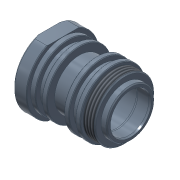
# Autodesk Inventor part: NA-45-h-Crown-307
Saved by Autodesk Inventor 2020.2 (Build 242310000, 310)
## iProperties
Created: 2020-04-21
Part Number: NA-45-h-Crown-307
Material: 14 100
Description: DRZAK CHYTAKU
Document SubType Name: Modeling
Designer: Jurek
Density: 7.85 g/cm^3
Mass: 123.312 g
Surface Area: 91.3308 cm^2
Volume: 15.7085 cm^3
Appearance: Ocelově modrá(1)
User Status: Rychlá změna
Checked By: Pippal
Category: B
Hmotnost (kg): 0,12
Rozmer_A: 36,7
Rozmer_B: 0
Rozmer_C: 0
Rozmer_D: 41
Rada vyrobku: 4100
Prumer nadobky: 45
Cislo artiklu: 4451101407
Jednotka: ks
Cisty rozmer: =Ø<Rozmer_A> - <Rozmer_D>
Predpona: Ø
Stroj na lince: Stahovací lis
RAZ Poznamka 1: ISO 2768-mH
RAZ Poznamka 2: NEOZNAČENÉ HRANY OJEHLIT
DXF: Ne
QAD_code: M
Rizeni davek: L
Author: Jurek
Revision Number: 00
Autodesk Inventor part; units mm, degrees
ref_plane "YZ Plane" through (0, 0, 0) normal (1, 0, 0) x (0, 1, 0)
ref_plane "XZ Plane" through (0, 0, 0) normal (0, 1, 0) x (-1, 0, 0)
ref_plane "XY Plane" through (0, 0, 0) normal (0, 0, 1) x (1, 0, 0)
sketch "Náčrt1" plane through (0, 0, 0) normal (0, 0, 1) x (1, 0, 0)
  line L0 (0, 0) -> (20.108, 0)
  line L1 (0, 12.5) -> (0, 18.35)
  line L2 (0, 18.35) -> (7, 18.35)
  line L3 (7, 18.35) -> (7, 16.35)
  line L4 (7, 16.35) -> (9.5, 16.35)
  line L5 (9.5, 16.35) -> (9.5, 14)
  line L6 (9.5, 14) -> (12.7, 14)
  line L7 (12.7, 14) -> (12.7, 16.35)
  line L8 (12.7, 16.35) -> (15.2, 16.35)
  line L9 (15.2, 16.35) -> (15.2, 12.5)
  line L10 (15.2, 12.5) -> (23.8, 12.5)
  line L11 (23.8, 12.5) -> (23.8, 16.35)
  line L12 (23.8, 16.35) -> (26.3, 16.35)
  line L13 (26.3, 16.35) -> (26.3, 14)
  line L14 (26.3, 14) -> (29.5, 14)
  line L15 (29.5, 14) -> (29.5, 16.35)
  line L16 (29.5, 16.35) -> (32, 16.35)
  line L17 (32, 16.35) -> (32, 15)
  line L18 (32, 15) -> (38, 15)
  line L19 (38, 15) -> (38, 12)
  line L20 (38, 12) -> (41, 12)
  line L21 (41, 12) -> (41, 10.2679)
  line L22 (40, 10) -> (34.5, 10)
  line L23 (33.567, 10.25) -> (10.933, 10.25)
  line L24 (10, 10) -> (2.5, 10)
  line L25 (34.5, 10) -> (33.567, 10.25)
  line L26 (10, 10) -> (10.933, 10.25)
  line L27 (0, 12.5) -> (2.5, 10)
  line L28 (40, 10) -> (41, 10.2679)
  dimension "d0" = 41
  dimension "d1" = 36.7
  dimension "d2" = 24
  dimension "d3" = 30
  dimension "d4" = 3
  dimension "d5" = 9
  dimension "d6" = 32.7
  dimension "d7" = 25
  dimension "d9" = 20
  dimension "d10" = 20
  dimension "d11" = 20.5
  dimension "d15" = 34
  dimension "d16" = 2.5
  dimension "d17" = 2.5
  dimension "d18" = 2.5
  dimension "d19" = 2.5
  dimension "d20" = 3.2
  dimension "d21" = 3.2
  dimension "d23" = 28
  dimension "d24" = 15
  dimension "d25" = 15
  dimension "d50" = 25
  dimension "d51" = 10
  dimension "d52" = 2.5
  dimension "d53" = 45
  dimension "d54" = 6.5
  dimension "d55" = 15
  dimension "d56" = 1
  constraints: 58 end point, 21 parallel, 5 point on line, 2 horizontal, 2 perpendicular
  measures "d0" distance between parallel lines of L21 L1
  measures "d1" diameter of L2 L0
  measures "d2" diameter of L20 L0
  measures "d3" diameter of L18 L0
  measures "d4" distance between parallel lines of L19 L21
  measures "d5" distance between parallel lines of L17 L21
  measures "d6" diameter of L16 L0
  measures "d7" diameter of L10 L0
  measures "d9" diameter of L24 L0
  measures "d10" diameter of L22 L0
  measures "d11" diameter of L23 L0
  measures "d15" distance between parallel lines of L3 L21
  measures "d16" distance between parallel lines of L15 L17
  measures "d17" distance between parallel lines of L11 L13
  measures "d18" distance between parallel lines of L7 L9
  measures "d19" distance between parallel lines of L5 L3
  measures "d20" distance between parallel lines of L15 L13
  measures "d21" distance between parallel lines of L7 L5
  measures "d23" diameter of L14 L0
  measures "d24" angle of L26 L24
  measures "d25" angle of L25 L22
  measures "d50" distance between parallel lines of L17 L3
  measures "d51" distance from line of L24.start L1
  measures "d52" distance from line of L24.end L1
  measures "d53" angle of L27 L24
  measures "d54" distance from line of L22.end L21
  measures "d55" angle of L28 L22
  measures "d56" distance from line of L22.start L21
revolve "Rotace1" add sketch "Náčrt1" angle 360 about axis through (0, 0, 0) along (1, 0, 0)
chamfer "Zkosení1" distance 1 angle 45 1 edges at (0, -18.35, 0)
chamfer "Zkosení2" distance 0.3 angle 45 1 edges at (7, -18.35, 0)
chamfer "Zkosení3" distance 0.5 angle 45 1 edges at (41, -12, 0)
chamfer "Zkosení4" distance 0.3 angle 45 7 edges at (32, -16.35, 0) (29.5, -16.35, 0) (26.3, -16.35, 0) (23.8, -16.35, 0) (15.2, -16.35, 0) (12.7, -16.35, 0) (9.5, -16.35, 0)
thread "Závit1" size "M30x1.5" class "6g" standard "ANSI Metric M Profile" full length
chamfer "Zkosení5" distance 0.5 angle 45 1 edges at (38, -15, 0)
sketch "Náčrt2" plane through (0, 0, 0) normal (-1, 0, 0) x (0, 0, 1)
  line L0 (-20.0207, 8.0295) -> (-16.5, 8.0295)
  line L1 (-16.5, 8.0295) -> (-16.5, -8.0295)
  line L2 (-16.5, -8.0295) -> (-20.0207, -8.0295)
  line L3 (-20.0207, -8.0295) -> (-20.0207, 8.0295)
  line L4 (28.0067, 8.0295) -> (16.5, 8.0295)
  line L5 (16.5, 8.0295) -> (16.5, -8.0295)
  line L6 (16.5, -8.0295) -> (28.0067, -8.0295)
  line L7 (28.0067, -8.0295) -> (28.0067, 8.0295)
  circle A0 centre (0, 0) radius 18.35 construction
  line L8 (0, 0) -> (0, 5.8894) construction
  dimension "d46" = 33
  constraints: 18 end point, 5 parallel, 2 horizontal, 2 perpendicular, 2 point on circle, 2 point on line, 1 other
  measures "d46" distance between parallel lines of L5 L1
extrude "Vysunutí1" cut sketch "Náčrt2" against normal through all
equation "\"d9\" = d10"
equation "\"Rozmer_A\" = d1"
equation "\"Rozmer_B\" = 0"
equation "\"Rozmer_C\" = 0"
equation "\"Rozmer_D\" = d0"
